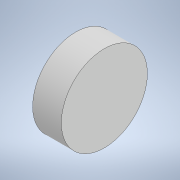
# Autodesk Inventor part: 711115
Saved by Autodesk Inventor 2022 (Build 260153000, 153)
## iProperties
Created: 2021-10-21
Part Number: 711115
Material: Типовые
Document SubType Name: Modeling
Designer: RaNSiD
Density: 1 g/cm^3
Appearance: По умолчанию
Mass: 56.3523 g
Surface Area: 95.8186 cm^2
Volume: 56.3523 cm^3
Author: RaNSiD
Autodesk Inventor part; units mm, degrees
ref_plane "YZ Plane" through (0, 0, 0) normal (1, 0, 0) x (0, 1, 0)
ref_plane "XZ Plane" through (0, 0, 0) normal (0, 1, 0) x (-1, 0, 0)
ref_plane "XY Plane" through (0, 0, 0) normal (0, 0, 1) x (1, 0, 0)
sketch "Эскиз1" plane through (0, 0, 0) normal (0, 0, 1) x (1, 0, 0)
  line L0 (0, 0) -> (20, 0)
  line L1 (20, 0) -> (20, 30)
  line L2 (20, 30) -> (0, 30)
  line L3 (0, 30) -> (0, 0)
  dimension "d0" = 20
  dimension "d1" = 30
  constraints: 8 end point, 2 parallel, 1 horizontal, 1 perpendicular
  measures "d0" distance of L2.end L1.end
  measures "d1" distance of L1.end L0.end
revolve "Вращение1" add sketch "Эскиз1" angle 360 about axis through (0, 0, 0) along (1, 0, 0)
sketch "Эскиз3" plane through (0, 0, 0) normal (0, 0, 1) x (1, 0, 0)
  line L0 (0, -30) -> (0, 30) construction
  line L1 (0, 26.5) -> (5, 26.5)
  line L2 (5, 26.5) -> (5, 21.5)
  line L3 (5, 21.5) -> (0, 21.5)
  line L4 (0, 21.5) -> (0, 26.5)
  line L5 (0, 18.5) -> (5, 18.5)
  line L6 (5, 18.5) -> (5, 13.5)
  line L7 (5, 13.5) -> (0, 13.5)
  line L8 (0, 13.5) -> (0, 18.5)
  line L9 (0, 0) -> (20, 0)
  line L10 (20, -30) -> (20, 30) projected
  dimension "d9" = 5
  dimension "d10" = 5
  dimension "d11" = 3
  dimension "d12" = 13.5
  constraints: 18 end point, 4 parallel, 2 horizontal, 2 midpoint, 2 perpendicular, 2 point on line, 1 collinear, 1 vertical alignment
  measures "d9" distance of L5.end L6.end
  measures "d10" distance of L6.end L7.end
  measures "d11" distance between parallel lines of L5 L3
  measures "d12" distance of point (0, 0) L7.end
revolve "Вращение2" cut sketch "Эскиз3" angle 360 about axis through (0, 0, 0) along (1, 0, 0)
